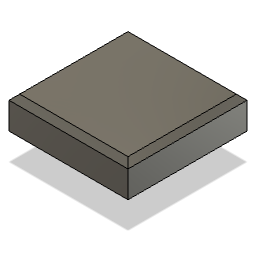
button v6 (Autodesk Fusion 360 design; units mm, degrees)
Autodesk Fusion 360 part; units mm, degrees
sketch "Sketch1" plane through (0, 0, 0) normal (0, 1, 0) x (1, 0, 0)
  line L0 (2.5299, -2.416) -> (-2.6613, -2.416)
  spline S0 degree 3 poles (-2.6613, -2.416) (-3.1243, -2.416) (-3.5, -2.0403) (-3.5, -1.5773) knots 0 0 0 0 1 1 1 1
  line L1 (-3.5, -1.5773) -> (-3.5, 1.5263)
  spline S1 degree 3 poles (-3.5, 1.5263) (-3.5, 1.9893) (-3.1243, 2.365) (-2.6613, 2.365) knots 0 0 0 0 1 1 1 1
  line L2 (-2.6613, 2.365) -> (-1.6082, 2.365)
  spline S2 degree 3 poles (-1.6082, 2.365) (-1.5183, 2.7301) (-1.1875, 3) (-0.7933, 3) knots 0 0 0 0 1 1 1 1
  line L3 (-0.7933, 3) -> (0.6778, 3)
  spline S3 degree 3 poles (0.6778, 3) (1.072, 3) (1.4054, 2.7301) (1.4927, 2.365) knots 0 0 0 0 1 1 1 1
  line L4 (1.4927, 2.365) -> (2.5272, 2.365)
  spline S4 degree 3 poles (2.5272, 2.365) (2.9902, 2.365) (3.3659, 1.9893) (3.3659, 1.5263) knots 0 0 0 0 1 1 1 1
  line L5 (3.3659, 1.5263) -> (3.3659, -1.5746)
  spline S5 degree 3 poles (3.3659, -1.5746) (3.3659, -2.0377) (2.9902, -2.4134) (2.5272, -2.4134) knots 0 0 0 0 1 1 1 1
  line L6 (2.5272, -2.4134) -> (2.5299, -2.416)
  spline S6 degree 3 poles (-0.0657, -1.5905) (-0.9283, -1.5905) (-1.632, -0.8867) (-1.632, -0.0242) knots 0 0 0 0 1 1 1 1
  spline S7 degree 3 poles (-1.632, -0.0242) (-1.632, 0.8384) (-0.9283, 1.5421) (-0.0657, 1.5421) knots 0 0 0 0 1 1 1 1
  spline S8 degree 3 poles (-0.0657, 1.5421) (0.7968, 1.5421) (1.5006, 0.8384) (1.5006, -0.0242) knots 0 0 0 0 1 1 1 1
  spline S9 degree 3 poles (1.5006, -0.0242) (1.5006, -0.8867) (0.7968, -1.5905) (-0.0657, -1.5905) knots 0 0 0 0 1 1 1 1
  spline S10 degree 3 poles (2.3235, 0.9998) (2.133, 0.9998) (1.9795, 1.1532) (1.9795, 1.3437) knots 0 0 0 0 1 1 1 1
  spline S11 degree 3 poles (1.9795, 1.3437) (1.9795, 1.5342) (2.133, 1.6877) (2.3235, 1.6877) knots 0 0 0 0 1 1 1 1
  spline S12 degree 3 poles (2.3235, 1.6877) (2.514, 1.6877) (2.6674, 1.5342) (2.6674, 1.3437) knots 0 0 0 0 1 1 1 1
  spline S13 degree 3 poles (2.6674, 1.3437) (2.6674, 1.1532) (2.514, 0.9997) (2.3235, 0.9998) knots 0 0 0 0 1 1 1 1
  line L7 (11.15, -11.15) -> (-11.15, -11.15)
  line L8 (-11.15, -11.15) -> (-11.15, 11.15)
  line L9 (-11.15, 11.15) -> (11.15, 11.15)
  line L10 (11.15, 11.15) -> (11.15, -11.15)
  line L11 (11.15, -11.15) -> (-11.15, 11.15) construction
  line L12 (-11.15, -11.15) -> (11.15, 11.15) construction
  line L13 (15, -15) -> (-15, -15)
  line L14 (-15, -15) -> (-15, 15)
  line L15 (-15, 15) -> (15, 15)
  line L16 (15, 15) -> (15, -15)
  line L17 (15, -15) -> (-15, 15) construction
  line L18 (-15, -15) -> (15, 15) construction
  dimension "d1" = 22.3
  dimension "d2" = 22.3
  dimension "d3" = 30
  dimension "d4" = 30
  constraint horizontal L7
  constraint perpendicular L7 L8
  constraint parallel L7 L9
  constraint parallel L8 L10
  constraint coincident L11 origin
  constraint coincident L12 origin
  constraint horizontal L13
  constraint perpendicular L13 L14
  constraint parallel L13 L15
  constraint parallel L14 L16
  constraint coincident L17 origin
  constraint coincident L18 origin
  measures "d1" distance of L8.end L9.end
  measures "d2" distance of L7.end L8.end
  measures "d3" distance of L14.end L15.end
  measures "d4" distance of L13.end L14.end
extrude "Extrude1" add sketch "Sketch1" against normal blind 5 contours L0 S0 L1 S1 L2 S2 L3 S3 L4 S4 L5 S5 L6 | S6 S7 S8 S9 | S10 S11 S12 S13 | L7 L8 L9 L10 makes body 1
extrude "Extrude2" cut sketch "Sketch1" against normal blind 0.5 contours L0 S0 L1 S1 L2 S2 L3 S3 L4 S4 L5 S5 L6 bodies 1
chamfer "Chamfer1" distance 1 angle 45 4 edges at (11.15, 0, 0) (0, 0, 11.15) (-11.15, 0, 0) (0, 0, -11.15) on bodies 1
sketch "Sketch2" plane through (0, -5, 0) normal (0, -1, 0) x (1, 0, 0)
  line L0 (-11.15, -11.15) -> (11.15, -11.15)
  line L1 (11.15, -11.15) -> (11.15, 11.15)
  line L2 (11.15, 11.15) -> (-11.15, 11.15)
  line L3 (-11.15, 11.15) -> (-11.15, -11.15)
  line L4 (3.25, 3.25) -> (-3.25, 3.25)
  line L5 (-3.25, 3.25) -> (-3.25, -3.25)
  line L6 (-3.25, -3.25) -> (3.25, -3.25)
  line L7 (3.25, -3.25) -> (3.25, 3.25)
  line L8 (3.25, 3.25) -> (-3.25, -3.25) construction
  line L9 (-3.25, 3.25) -> (3.25, -3.25) construction
  dimension "d10" = 6.5
  dimension "d11" = 6.5
  constraint horizontal L4
  constraint perpendicular L4 L5
  constraint parallel L4 L6
  constraint parallel L5 L7
  constraint coincident L8 origin
  constraint coincident L9 origin
  measures "d10" distance of L5.end L6.end
  measures "d11" distance of L4.end L5.end
sketch "Sketch3" plane through (0, -5, 0) normal (0, -1, 0) x (1, 0, 0)
  line L0 (0.585, 2.05) -> (-0.585, 2.05)
  line L1 (-0.585, 2.05) -> (-0.585, -2.05)
  line L2 (-0.585, -2.05) -> (0.585, -2.05)
  line L3 (0.585, -2.05) -> (0.585, 2.05)
  line L4 (0.585, 2.05) -> (-0.585, -2.05) construction
  line L5 (-0.585, 2.05) -> (0.585, -2.05) construction
  line L6 (2.05, -0.585) -> (-2.05, -0.585)
  line L7 (-2.05, -0.585) -> (-2.05, 0.585)
  line L8 (-2.05, 0.585) -> (2.05, 0.585)
  line L9 (2.05, 0.585) -> (2.05, -0.585)
  line L10 (2.05, -0.585) -> (-2.05, 0.585) construction
  line L11 (-2.05, -0.585) -> (2.05, 0.585) construction
  line L12 (1.2, -2.7) -> (-1.2, -2.7)
  line L13 (-2.7, -1.2) -> (-2.7, 1.2)
  line L14 (-1.2, 2.7) -> (1.2, 2.7)
  line L15 (2.7, 1.2) -> (2.7, -1.2)
  line L16 (2.7, -2.7) -> (-2.7, 2.7) construction
  line L17 (-2.7, -2.7) -> (2.7, 2.7) construction
  arc A0 (-1.2, 2.7) -> (-2.7, 1.2) centre (-1.2, 1.2) ccw
  arc A1 (2.7, 1.2) -> (1.2, 2.7) centre (1.2, 1.2) ccw
  arc A2 (1.2, -2.7) -> (2.7, -1.2) centre (1.2, -1.2) ccw
  arc A3 (-2.7, -1.2) -> (-1.2, -2.7) centre (-1.2, -1.2) ccw
  line L18 (-2.25, 0.785) -> (2.25, 0.785)
  line L19 (2.25, 0.785) -> (2.25, -0.785)
  line L20 (2.25, -0.785) -> (-2.25, -0.785)
  line L21 (-2.25, -0.785) -> (-2.25, 0.785)
  line L22 (0.785, -2.25) -> (0.785, 2.25)
  line L23 (0.785, 2.25) -> (-0.785, 2.25)
  line L24 (-0.785, 2.25) -> (-0.785, -2.25)
  line L25 (-0.785, -2.25) -> (0.785, -2.25)
  dimension "d12" = 1.17
  dimension "d13" = 4.1
  dimension "d14" = 4.1
  dimension "d15" = 1.17
  dimension "d16" = 5.4
  dimension "d17" = 5.4
  dimension "d18" = 1.5
  dimension "d19" = 1.5
  dimension "d20" = 1.5
  dimension "d21" = 1.5
  dimension "d35" = -0.2
  dimension "d36" = 0.2
  constraint horizontal L0
  constraint perpendicular L0 L1
  constraint parallel L0 L2
  constraint parallel L1 L3
  constraint coincident L4 origin
  constraint coincident L5 origin
  constraint horizontal L6
  constraint perpendicular L6 L7
  constraint parallel L6 L8
  constraint parallel L7 L9
  constraint coincident L10 origin
  constraint coincident L11 origin
  constraint horizontal L12
  constraint perpendicular L12 L13
  constraint parallel L12 L14
  constraint parallel L13 L15
  constraint coincident L16 origin
  constraint coincident L17 origin
  constraint coincident L16.end L14
  constraint coincident L16.end L13
  constraint tangent L14 A0
  constraint tangent L13 A0
  constraint coincident L17.end L15
  constraint coincident L17.end L14
  constraint tangent L15 A1
  constraint tangent L14 A1
  constraint coincident L16.start L15
  constraint coincident L16.start L12
  constraint tangent L15 A2
  constraint tangent L12 A2
  constraint coincident L17.start L13
  constraint coincident L17.start L12
  constraint tangent L13 A3
  constraint tangent L12 A3
  measures "d12" distance of L1.end L2.end
  measures "d13" distance of L0.end L1.end
  measures "d14" distance of L7.end L8.end
  measures "d15" distance of L6.end L7.end
  measures "d16" distance of L16.end L17.end
  measures "d17" distance of L17.start L16.end
  measures "d18" radius of A0
  measures "d19" radius of A1
  measures "d20" radius of A2
  measures "d21" radius of A3
extrude "Extrude3" add sketch "Sketch3" along normal blind 3 contours L0 L1 L3 L18 L22 L23 L24 | L3 L8 L18 L22 | L1 L8 L18 L24 | L6 L8 L9 L18 L19 L20 L22 | L6 L7 L8 L18 L20 L21 L24 | L3 L6 L20 L22 | L1 L6 L20 L24 | L1 L2 L3 L20 L22 L24 L25 | L12 L13 L14 L15 A0 A1 A2 A3 bodies 1
chamfer "Chamfer2" distance 1 angle 45 1 faces at (-8.3333, -5, 0.4) on bodies 1
move_face "MoveFace1" by (0, -1, 0) 1 faces at (-1.6058, -8, 1.6562) on bodies 1
extrude "Extrude4" add sketch "Sketch1" against normal blind 3 separate body contours L0 S0 L1 S1 L2 S2 L3 S3 L4 S4 L5 S5 L6 | S6 S7 S8 S9 | S10 S11 S12 S13 | L7 L8 L9 L10 | L13 L14 L15 L16 makes body 2
extrude "Extrude5" add sketch "Sketch1" against normal blind 7 contours L0 S0 L1 S1 L2 S2 L3 S3 L4 S4 L5 S5 L6 | S6 S7 S8 S9 | S10 S11 S12 S13 | L7 L8 L9 L10 bodies 2
extrude "Extrude6" cut sketch "Sketch1" against normal blind 0.5 contours L0 S0 L1 S1 L2 S2 L3 S3 L4 S4 L5 S5 L6 bodies 2
extrude "Extrude7" add sketch "Sketch3" along normal blind 5 contours L0 L1 L3 L18 L22 L23 L24 | L3 L8 L18 L22 | L1 L8 L18 L24 | L6 L8 L9 L18 L19 L20 L22 | L6 L7 L8 L18 L20 L21 L24 | L3 L6 L20 L22 | L1 L6 L20 L24 | L1 L2 L3 L20 L22 L24 L25 | L12 L13 L14 L15 A0 A1 A2 A3 bodies 2
move_face "MoveFace2" by (0, 2, 0) 5 faces at (0.8433, 0, 7.572) (10.8167, -0.6667, 3.3833) (-3.3833, -0.6667, 10.8167) (3.3833, -0.6667, -10.8167) (-10.8167, -0.6667, 3.3833) on bodies 1
extrude "Extrude8" add 2 faces at (2.3235, 0, -1.4584) (-0.1493, 0, 0.6549) along direction (0, 1, 0) blind 2 on bodies 1 bodies 1
extrude "Extrude9" cut sketch "Sketch3" along normal blind 4.4 contours L0 L1 L3 L18 | L0 L1 L3 L18 L22 L23 L24 | L3 L8 L18 L22 | L1 L3 L8 L18 | L1 L8 L18 L24 | L3 L6 L8 L22 | L1 L3 L6 L8 | L6 L8 L9 L18 L19 L20 L22 | L1 L6 L8 L24 | L6 L7 L8 L18 L20 L21 L24 | L3 L6 L20 L22 | L1 L3 L6 L20 | L6 L8 L9 L22 | L1 L6 L20 L24 | L6 L7 L8 L24 | L1 L2 L3 L20 L22 L24 L25 | L1 L2 L3 L20 bodies 1
sketch "Sketch4" plane through (0, -0.5, 0) normal (0, 1, 0) x (-1, 0, 0)
  spline S0 degree 3 poles (-2.6674, -1.3437) (-2.6674, -1.5342) (-2.514, -1.6877) (-2.3235, -1.6877) knots -1 -1 -1 -1 0 0 0 0
  spline S1 degree 3 poles (-2.3235, -0.9998) (-2.514, -0.9997) (-2.6674, -1.1532) (-2.6674, -1.3437) knots -1 -1 -1 -1 0 0 0 0
  spline S2 degree 3 poles (-1.9795, -1.3437) (-1.9795, -1.1532) (-2.133, -0.9998) (-2.3235, -0.9998) knots -1 -1 -1 -1 0 0 0 0
  spline S3 degree 3 poles (-2.3235, -1.6877) (-2.133, -1.6877) (-1.9795, -1.5342) (-1.9795, -1.3437) knots -1 -1 -1 -1 0 0 0 0
  spline S4 degree 3 poles (-1.5006, 0.0242) (-1.5006, -0.8384) (-0.7968, -1.5421) (0.0657, -1.5421) knots -1 -1 -1 -1 0 0 0 0
  spline S5 degree 3 poles (0.0657, 1.5905) (-0.7968, 1.5905) (-1.5006, 0.8867) (-1.5006, 0.0242) knots -1 -1 -1 -1 0 0 0 0
  spline S6 degree 3 poles (1.632, 0.0242) (1.632, 0.8867) (0.9283, 1.5905) (0.0657, 1.5905) knots -1 -1 -1 -1 0 0 0 0
  spline S7 degree 3 poles (0.0657, -1.5421) (0.9283, -1.5421) (1.632, -0.8384) (1.632, 0.0242) knots -1 -1 -1 -1 0 0 0 0
  spline S8 degree 3 poles (-3.3659, 1.5746) (-3.3659, 2.0377) (-2.9902, 2.4134) (-2.5272, 2.4134) knots 0 0 0 0 1 1 1 1
  line L0 (-3.3659, 1.5746) -> (-3.3659, -1.5263)
  spline S9 degree 3 poles (-2.5272, -2.365) (-2.9902, -2.365) (-3.3659, -1.9893) (-3.3659, -1.5263) knots 0 0 0 0 1 1 1 1
  line L1 (-2.5272, -2.365) -> (-1.4927, -2.365)
  spline S10 degree 3 poles (-0.6778, -3) (-1.072, -3) (-1.4054, -2.7301) (-1.4927, -2.365) knots 0 0 0 0 1 1 1 1
  line L2 (-0.6778, -3) -> (0.7933, -3)
  spline S11 degree 3 poles (1.6082, -2.365) (1.5183, -2.7301) (1.1875, -3) (0.7933, -3) knots 0 0 0 0 1 1 1 1
  line L3 (1.6082, -2.365) -> (2.6613, -2.365)
  spline S12 degree 3 poles (3.5, -1.5263) (3.5, -1.9893) (3.1243, -2.365) (2.6613, -2.365) knots 0 0 0 0 1 1 1 1
  line L4 (3.5, -1.5263) -> (3.5, 1.5773)
  spline S13 degree 3 poles (2.6613, 2.416) (3.1243, 2.416) (3.5, 2.0403) (3.5, 1.5773) knots 0 0 0 0 1 1 1 1
  line L5 (2.6613, 2.416) -> (-2.5299, 2.416)
  line L6 (-2.5299, 2.416) -> (-2.5272, 2.4134)
sketch "Sketch5" plane through (0, 2, 0) normal (0, 1, 0) x (-1, 0, 0)
  line L0 (-4.1435, -1.8722) -> (-4.1435, 1.9233)
  spline S0 degree 3 poles (-4.1435, 1.9233) (-4.1435, 1.9947) (-4.1362, 2.0657) (-4.1073, 2.2033) (-4.0862, 2.2694) (-4.0045, 2.4568) (-3.9263, 2.5688) (-3.7345, 2.7536) (-3.6234, 2.826) (-3.3792, 2.9248) (-3.2492, 2.9498) (-3.117, 2.9498) knots -0.132389 -0.132389 -0.132389 -0.132389 -0.114861 -0.114861 -0.097861 -0.097861 -0.064668 -0.064668 -0.032414 -0.032414 0 0 0 0
  line L1 (-3.117, 2.9498) -> (-3.1202, 2.9531)
  line L2 (-3.1202, 2.9531) -> (3.2336, 2.9531)
  spline S1 degree 3 poles (3.2336, 2.9531) (3.305, 2.9531) (3.376, 2.9458) (3.5137, 2.9168) (3.5797, 2.8957) (3.7671, 2.814) (3.8791, 2.7358) (4.0639, 2.544) (4.1363, 2.4329) (4.2351, 2.1888) (4.2602, 2.0587) (4.2602, 1.9265) knots -0.132389 -0.132389 -0.132389 -0.132389 -0.114861 -0.114861 -0.097861 -0.097861 -0.064668 -0.064668 -0.032414 -0.032414 0 0 0 0
  line L3 (4.2602, 1.9265) -> (4.2602, -1.8722)
  spline S2 degree 3 poles (4.2602, -1.8722) (4.2602, -1.9436) (4.2529, -2.0146) (4.2239, -2.1523) (4.2028, -2.2183) (4.1211, -2.4057) (4.0429, -2.5177) (3.8511, -2.7025) (3.74, -2.7749) (3.4958, -2.8737) (3.3658, -2.8988) (3.2336, -2.8988) knots -0.132389 -0.132389 -0.132389 -0.132389 -0.114861 -0.114861 -0.097861 -0.097861 -0.064668 -0.064668 -0.032414 -0.032414 0 0 0 0
  line L4 (3.2336, -2.8988) -> (1.9447, -2.8988)
  spline S3 degree 3 poles (1.9447, -2.8988) (1.9217, -2.9921) (1.8855, -3.0815) (1.7899, -3.2465) (1.7312, -3.3214) (1.5686, -3.4786) (1.4572, -3.5512) (1.2118, -3.6507) (1.0806, -3.676) (0.9473, -3.676) knots -0.111889 -0.111889 -0.111889 -0.111889 -0.088278 -0.088278 -0.06503 -0.06503 -0.032688 -0.032688 0 0 0 0
  line L5 (0.9473, -3.676) -> (-0.8533, -3.676)
  spline S4 degree 3 poles (-0.8533, -3.676) (-0.9538, -3.676) (-1.0534, -3.6616) (-1.2426, -3.6053) (-1.331, -3.5647) (-1.5233, -3.4411) (-1.6196, -3.3491) (-1.7684, -3.1381) (-1.8213, -3.022) (-1.8507, -2.8988) knots -0.111741 -0.111741 -0.111741 -0.111741 -0.087119 -0.087119 -0.063358 -0.063358 -0.031063 -0.031063 0 0 0 0
  line L6 (-1.8507, -2.8988) -> (-3.117, -2.8988)
  spline S5 degree 3 poles (-3.117, -2.8988) (-3.1884, -2.8988) (-3.2594, -2.8915) (-3.3971, -2.8625) (-3.4631, -2.8414) (-3.6505, -2.7597) (-3.7625, -2.6815) (-3.9473, -2.4897) (-4.0197, -2.3786) (-4.1185, -2.1344) (-4.1435, -2.0044) (-4.1435, -1.8722) knots -0.132389 -0.132389 -0.132389 -0.132389 -0.114861 -0.114861 -0.097861 -0.097861 -0.064668 -0.064668 -0.032414 -0.032414 0 0 0 0
  line L7 (12.3996, 12.4192) -> (-12.447, 12.4192)
  line L8 (-12.447, 12.4192) -> (-12.447, -12.4274)
  line L9 (-12.447, -12.4274) -> (12.3996, -12.4274)
  line L10 (12.3996, -12.4274) -> (12.3996, 12.4192)
  spline S6 degree 3 poles (-4.1435, 1.9233) (-4.1435, 1.9947) (-4.1362, 2.0657) (-4.1073, 2.2033) (-4.0862, 2.2694) (-4.0045, 2.4568) (-3.9263, 2.5688) (-3.7345, 2.7536) (-3.6234, 2.826) (-3.3792, 2.9248) (-3.2492, 2.9498) (-3.117, 2.9498) knots -0.132389 -0.132389 -0.132389 -0.132389 -0.114861 -0.114861 -0.097861 -0.097861 -0.064668 -0.064668 -0.032414 -0.032414 0 0 0 0
  spline S7 degree 3 poles (4.2602, -1.8722) (4.2602, -1.9436) (4.2529, -2.0146) (4.2239, -2.1523) (4.2028, -2.2183) (4.1211, -2.4057) (4.0429, -2.5177) (3.8511, -2.7025) (3.74, -2.7749) (3.4958, -2.8737) (3.3658, -2.8988) (3.2336, -2.8988) knots -0.132389 -0.132389 -0.132389 -0.132389 -0.114861 -0.114861 -0.097861 -0.097861 -0.064668 -0.064668 -0.032414 -0.032414 0 0 0 0
  line L11 (-3.117, 2.9498) -> (-3.1202, 2.9531)
  spline S8 degree 3 poles (-0.8533, -3.676) (-0.9538, -3.676) (-1.0534, -3.6616) (-1.2426, -3.6053) (-1.331, -3.5647) (-1.5233, -3.4411) (-1.6196, -3.3491) (-1.7684, -3.1381) (-1.8213, -3.022) (-1.8507, -2.8988) knots -0.111741 -0.111741 -0.111741 -0.111741 -0.087119 -0.087119 -0.063358 -0.063358 -0.031063 -0.031063 0 0 0 0
  spline S9 degree 3 poles (1.9447, -2.8988) (1.9217, -2.9921) (1.8855, -3.0815) (1.7899, -3.2465) (1.7312, -3.3214) (1.5686, -3.4786) (1.4572, -3.5512) (1.2118, -3.6507) (1.0806, -3.676) (0.9473, -3.676) knots -0.111889 -0.111889 -0.111889 -0.111889 -0.088278 -0.088278 -0.06503 -0.06503 -0.032688 -0.032688 0 0 0 0
  line L12 (3.2336, -2.8988) -> (1.9447, -2.8988)
  spline S10 degree 3 poles (3.2336, 2.9531) (3.305, 2.9531) (3.376, 2.9458) (3.5137, 2.9168) (3.5797, 2.8957) (3.7671, 2.814) (3.8791, 2.7358) (4.0639, 2.544) (4.1363, 2.4329) (4.2351, 2.1888) (4.2602, 2.0587) (4.2602, 1.9265) knots -0.132389 -0.132389 -0.132389 -0.132389 -0.114861 -0.114861 -0.097861 -0.097861 -0.064668 -0.064668 -0.032414 -0.032414 0 0 0 0
  line L13 (-12.447, 12.4192) -> (-12.447, -12.4274)
  line L14 (-3.1202, 2.9531) -> (3.2336, 2.9531)
  line L15 (0.9473, -3.676) -> (-0.8533, -3.676)
  line L16 (4.2602, 1.9265) -> (4.2602, -1.8722)
  spline S11 degree 3 poles (-3.117, -2.8988) (-3.1884, -2.8988) (-3.2594, -2.8915) (-3.3971, -2.8625) (-3.4631, -2.8414) (-3.6505, -2.7597) (-3.7625, -2.6815) (-3.9473, -2.4897) (-4.0197, -2.3786) (-4.1185, -2.1344) (-4.1435, -2.0044) (-4.1435, -1.8722) knots -0.132389 -0.132389 -0.132389 -0.132389 -0.114861 -0.114861 -0.097861 -0.097861 -0.064668 -0.064668 -0.032414 -0.032414 0 0 0 0
  line L17 (-1.8507, -2.8988) -> (-3.117, -2.8988)
  line L18 (-4.1435, -1.8722) -> (-4.1435, 1.9233)
  circle A0 centre (-2.8651, -1.6732) radius 0.612
  circle A1 centre (0.3523, -0.0041) radius 2.1419
  point P0 (-0.0237, -0.0041)
  point P1 (0.106, 0.0181)
  dimension "d40" = 1
  dimension "d44" = 3.5
scale "Scale1" [no effect]
extrude "Extrude10" add 1 faces at (-2.8773, -0.5, 0.0251) along direction (0, 1, 0) blind 2.5 on bodies 1 bodies 1
extrude "Extrude11" cut sketch "Sketch5" against normal blind 2 contours L0 S0 L1 L2 S1 L3 S2 L4 S3 L5 S4 L6 S5 S6 S7 L11 S8 S9 L12 S10 L14 L15 L16 S11 L17 L18 bodies 1
extrude "Extrude12" add 1 faces at (-3.6715, 0, 0.0168) along direction (0, 1, 0) blind 2 on bodies 1 bodies 1
hidden bodies 2
